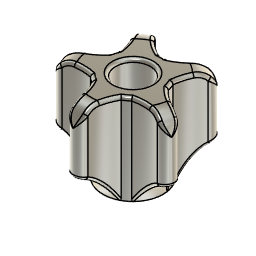
GPS_KNOB (Autodesk Fusion 360 design; units mm, degrees)
Autodesk Fusion 360 part; units mm, degrees
sketch "Esquisse1" plane through (0, 0, 0) normal (0, 0, 1) x (1, 0, 0)
  circle A0 centre (0, 0) radius 2.9
  line L0 (0, 0) -> (0, -10) construction
  line L1 (0, 0) -> (0, 7) construction
  circle A1 centre (0, 5.75) radius 1.25 construction
  circle A2 centre (0, -8.75) radius 1.25 construction
  line L2 (0, 5.75) -> (-1.25, 5.75) construction
  line L3 (0, -8.75) -> (-1.25, -8.75) construction
  line L4 (0, -8.75) -> (1.25, -8.75) construction
  line L5 (0, 5.75) -> (1.25, 5.75) construction
  circle A3 centre (0, 0) radius 5
  arc A4 (-1.25, -8.75) -> (1.25, -8.75) centre (0, -8.75) ccw
  arc A5 (-1.25, -8.75) -> (-2.408218, -4.381836) centre (-10.06627, -8.75) ccw
  arc A6 (2.408218, -4.381836) -> (1.25, -8.75) centre (10.06627, -8.75) ccw
  arc A7 (7.935473, -3.892719) -> (3.423193, -3.644413) centre (5.211096, -12.27749) ccw
  arc A8 (7.935473, -3.892719) -> (8.708016, -1.515078) centre (8.321745, -2.703899) ccw
  arc A9 (4.911554, 0.93629) -> (8.708016, -1.515078) centre (11.432393, 6.869693) ccw
  arc A10 (6.154392, 6.344167) -> (4.523868, 2.129465) centre (13.286904, 1.162094) ccw
  arc A11 (6.154392, 6.344167) -> (4.13185, 7.81363) centre (5.143121, 7.078899) ccw
  arc A12 (0.627289, 4.960495) -> (4.13185, 7.81363) centre (-3.000662, 12.995704) ccw
  arc A13 (-4.13185, 7.81363) -> (-0.627289, 4.960495) centre (3.000662, 12.995704) ccw
  arc A14 (-4.13185, 7.81363) -> (-6.154392, 6.344167) centre (-5.143121, 7.078899) ccw
  arc A15 (-4.523868, 2.129465) -> (-6.154392, 6.344167) centre (-13.286904, 1.162094) ccw
  arc A16 (-8.708016, -1.515078) -> (-4.911554, 0.93629) centre (-11.432393, 6.869693) ccw
  arc A17 (-8.708016, -1.515078) -> (-7.935473, -3.892719) centre (-8.321745, -2.703899) ccw
  arc A18 (-3.423193, -3.644413) -> (-7.935473, -3.892719) centre (-5.211096, -12.27749) ccw
  dimension "d1" = 5.8
  dimension "d2" = 10
  dimension "d3" = 2.5
  dimension "d4" = 1.25
  dimension "d5" = 2.5
  dimension "d6" = 10
  dimension "d27" = 360
  constraint coincident A0.centre L0.start
  constraint vertical L0
  constraint parallel L0 L1
  constraint coincident L1 A1.centre
  constraint coincident L1.end A1
  constraint coincident L0 A2.centre
  constraint coincident A1.centre L2.start
  constraint coincident A1 L2.end
  constraint perpendicular L1 L2
  constraint coincident A2.centre L3.start
  constraint coincident A2 L3.end
  constraint perpendicular L0 L3
  constraint coincident A2 L4.end
  constraint perpendicular L0 L4
  constraint coincident A1 L5.end
  constraint parallel L4 L5
  constraint concentric A0 A3
  constraint tangent A2 A5
  constraint symmetric L0 L3.end L4.end
  constraint symmetric L0 A5 A6
  measures "d1" diameter of A0
  measures "d2" distance of A0.centre L0.end
  measures "d3" diameter of A2
  measures "d4" distance of L0.end A2.centre
  measures "d5" diameter of A1
  measures "d6" diameter of A3
extrude "Extrusion1" add sketch "Esquisse1" along normal blind 15 contours A3 | A3 A7 A8 A9 | A3 A10 A11 A12 | A3 A4 A5 A6 | A3 A13 A14 A15 | A3 A16 A17 A18 picked at (-3.540252, -2.425454) picked at (5.720477, -1.785238) picked at (3.423729, 4.915744) picked at (-0.119547, -5.989338) picked at (-3.423729, 4.915744) picked at (-5.733141, -1.737111)
sketch "Esquisse4" plane through (0, 0, 0) normal (1, 0, 0) x (0, 1, 0)
  line L0 (0, 0) -> (-5, 0)
  line L1 (-5, 0) -> (-10, 0)
  line L2 (-10, 0) -> (-10, 5)
  line L3 (-10, 5) -> (-10, 12)
  line L4 (0, 15) -> (-7, 15)
  arc A0 (-7, 15) -> (-10, 12) centre (-7, 12) ccw
  arc A1 (-5, 0) -> (-10, 5) centre (-12.795656, -2.795656) ccw
  line L5 (-5, 0) -> (-10, 0)
  line L6 (-10, 0) -> (-10, 5)
  line L7 (-7, 15) -> (-10, 15)
  line L8 (-10, 15) -> (-10, 12)
  line L9 (0, 15) -> (0, 0)
  dimension "d28" = 5
  dimension "d29" = 5
  dimension "d30" = 7
  dimension "d31" = 7
  constraint coincident L0.start L9.end
  constraint horizontal L0
  constraint parallel L0 L1
  constraint perpendicular L1 L2
  constraint parallel L2 L3
  constraint horizontal L4
  constraint tangent L3 A0
  constraint tangent A0 L7
  constraint tangent A0 L8
  constraint perpendicular L0 L9
  measures "d28" distance of L0.start L0.end
  measures "d29" distance of L1.end L2.end
  measures "d30" distance of L2.end L3.end
  measures "d31" distance of L4.start L4.end
revolve "Révolution2" cut sketch "Esquisse4" angle 360 about axis through (0, 0, 15) along (0, 0, -1) contours L1 L2 A1 L5 L6 | A0 L7 L8 picked at (-8.26672, 2.305201) picked at (-9.41061, 14.41061)
fillet "Congé5" radius 0.5 35 edges at (-4.957019, 8.31499, 13.347359) (-3.563078, 7.109799, 14.844723) (-1.790089, 5.594669, 15) (-4.767678, 3.431324, 15) (-5.67431, 5.60899, 14.835896) (-6.376223, 7.283878, 13.347359) (-5.874014, 0.026372, 15) (-7.894039, -1.205367, 14.833502) (-9.441705, -2.148711, 13.342022) (-4.736676, -3.473994, 15) (-7.093512, -3.664537, 14.833986) (-8.901481, -3.811351, 13.342022) (-4.755283, 1.545085, 15) (-2.938926, -4.045085, 15) (-1.840251, -5.57837, 15) (-1.293098, -7.879338, 14.833777) (-0.840426, -9.67532, 13.283093) (1.840251, -5.57837, 15) (1.296548, -7.84525, 14.845056) (0.840426, -9.67532, 13.283093) (2.938926, -4.045085, 15) (4.736676, -3.473994, 15) (7.095168, -3.664893, 14.833412) (8.901481, -3.811351, 13.342022) (5.874014, 0.026372, 15) (7.891759, -1.204363, 14.834342) (9.441705, -2.148711, 13.342022) (4.755283, 1.545085, 15) (4.767678, 3.431324, 15) (5.660769, 5.585737, 14.844724) (6.376223, 7.283878, 13.347359) (1.790089, 5.594669, 15) (3.581116, 7.129983, 14.835842) (4.957019, 8.31499, 13.347359) (0, 5, 15)
fillet "Congé6" radius 0.5 21 edges at (-2.703749, 1.048685, 15) (-2.362333, 5.998007, 2.521767) (-4.91636, 8.308161, 4.867034) (-6.382344, 7.242713, 4.866925) (-4.976258, 4.105765, 2.527595) (4.974443, 4.100198, 2.521768) (6.382292, 7.243099, 4.867034) (4.915977, 8.308091, 4.866925) (2.367064, 6.00145, 2.527589) (5.436822, -3.463851, 2.521797) (8.860271, -3.831948, 4.866862) (9.420743, -2.108323, 4.867014) (6.435212, -0.393635, 2.522739) (-1.614655, -6.2394, 2.519915) (-0.90599, -9.611212, 4.867036) (0.90577, -9.611441, 4.867121) (1.613528, -6.242045, 2.522556) (-6.434449, -0.393299, 2.521763) (-9.420472, -2.107826, 4.866862) (-8.860782, -3.831705, 4.867014) (-5.437076, -3.464045, 2.522228)
